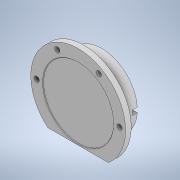
# Autodesk Inventor part: 轴承端盖3
Saved by Autodesk Inventor 2020 (Build 240168000, 168)
## iProperties
Created: 2021-06-16
Part Number: 轴承端盖3
Material: 常规
Document SubType Name: Modeling
Designer: dell
Density: 1 g/cm^3
Appearance: 默认
Author: dell
Autodesk Inventor part; units mm, degrees
ref_plane "YZ Plane" through (0, 0, 0) normal (1, 0, 0) x (0, 1, 0)
ref_plane "XZ Plane" through (0, 0, 0) normal (0, 1, 0) x (-1, 0, 0)
ref_plane "XY Plane" through (0, 0, 0) normal (0, 0, 1) x (1, 0, 0)
ref_plane "工作平面1" through (0, 0, 0) normal (0, 0, 1) x (1, 0, 0)
sketch "草图1" plane through (0, 0, 0) normal (0, 0, 1) x (1, 0, 0)
  arc A0 (9.993, -85.0026) -> (-35, 93.8712) centre (-50, -4.9974) ccw construction
  arc A1 (-50, -79.9974) -> (-50, 70.0026) centre (-50, -4.9974) ccw construction
  line L0 (-50, -79.9974) -> (-50, -85.0026) construction
  line L1 (-35, -85.0026) -> (-50, -85.0026) construction
  line L2 (-35, -95.0026) -> (-35, -85.0026) construction
  line L3 (9.993, -95.0026) -> (-35, -95.0026) construction
  line L4 (9.993, -95.0026) -> (9.993, -85.0026) construction
  arc A2 (9.993, -85.0026) -> (-35, 93.8712) centre (-50, -4.9974) ccw construction
  line L5 (-35, 93.8712) -> (-35, 95.0026) construction
  line L6 (-35, 95.0026) -> (-50, 95.0026) construction
  line L7 (-50, 95.0026) -> (-50, 70.0026) construction
  arc A3 (13.8044, -81.9974) -> (-113.8044, -81.9974) centre (-50, -4.9974) ccw
  line L8 (-113.8044, -81.9974) -> (13.8044, -81.9974)
  circle A4 centre (-50, -4.9974) radius 87.5 construction
  line L9 (-162.5015, -4.9974) -> (70.6652, -4.9974) construction
  circle A5 centre (-137.5, -4.9974) radius 5.5
  circle A6 centre (-93.75, -80.7746) radius 5.5 construction
  circle A7 centre (-6.25, -80.7746) radius 5.5 construction
  circle A8 centre (37.5, -4.9974) radius 5.5
  circle A9 centre (-6.25, 70.7799) radius 5.5
  circle A10 centre (-93.75, 70.7799) radius 5.5
  point P0 (0, 0)
  point P1 (-50, -81.9974)
  dimension "d1" = 175
  dimension "d0" = 2
  dimension "d2" = 11
  dimension "d5" = 360
  constraints: 7 centre point, 4 end point, 3 point on line, 2 coincident, 2 horizontal, 2 point on circle, 1 concentric, 1 horizontal alignment, 1 midpoint, 15 other
  measures "d0" distance of L0.start point (-50, -81.997)
  measures "d2" diameter of A5
extrude "拉伸1" add sketch "草图1" along normal blind 12
sketch "草图2" plane through (0, 0, 0) normal (0, 0, -1) x (-1, 0, 0)
  arc A0 (113.8044, -81.9974) -> (-13.8044, -81.9974) centre (50, -4.9974) ccw construction
  circle A1 centre (50, -4.9974) radius 75
  circle A2 centre (50, -4.9974) radius 65
  point P0 (0, 0)
  dimension "d9" = 150
  dimension "d10" = 10
  constraints: 2 centre point, 1 coincident
  measures "d9" diameter of A1
  measures "d10" radial gap between concentric circles of A1 A2
extrude "拉伸2" add sketch "草图2" along normal blind 38
sketch "草图3" plane through (0, 0, 12) normal (0, 0, 1) x (1, 0, 0)
  arc A0 (13.8044, -81.9974) -> (-113.8044, -81.9974) centre (-50, -4.9974) ccw construction
  circle A1 centre (-50, -4.9974) radius 75
  circle A2 centre (-137.5, -4.9974) radius 5.5 construction
  point P0 (0, 0)
  dimension "d13" = 150
  constraints: 1 centre point, 1 coincident
  measures "d13" diameter of A1
extrude "拉伸3" cut sketch "草图3" against normal blind 1
fillet "圆角1" radius 1 1 edges at (-125, -4.9974, 11)
sketch "草图4" plane through (-50, -4.9974, -38) normal (0, 0, -1) x (-1, 0, 0)
  line L0 (100, 5) -> (-100, 5)
  line L1 (-100, 5) -> (-100, -5)
  line L2 (-100, -5) -> (100, -5)
  line L3 (100, -5) -> (100, 5)
  circle A0 centre (0, 0) radius 65 construction
  point P0 (-50, 4.9974)
  point P1 (100, 0)
  point P2 (0, -5)
  dimension "d17" = 10
  dimension "d18" = 200
  constraints: 8 end point, 2 midpoint, 2 parallel, 1 horizontal, 1 horizontal alignment, 1 perpendicular, 1 vertical alignment
  measures "d17" distance between parallel lines of L2 L0
  measures "d18" distance of L1.end L2.end
extrude "拉伸4" cut sketch "草图4" against normal blind 10
sketch "草图5" plane through (-50, -4.9974, 0) normal (0, 0, -1) x (-1, 0, 0)
  circle A0 centre (0, 0) radius 65 projected
  point P0 (-50, 4.9974)
extrude "拉伸5" add sketch "草图5" along normal blind 3
